foam_v5 (Autodesk Fusion 360 design; units mm, degrees)
Autodesk Fusion 360 part; units mm, degrees
sketch "Sketch1" plane through (0, 0, 0) normal (0, 1, 0) x (1, 0, 0)
  line L0 (0, 0) -> (215.9, 0)
  line L1 (215.9, 0) -> (215.9, 106.3625) construction
  line L2 (215.9, 106.3625) -> (0, 106.3625) construction
  line L3 (0, 106.3625) -> (0, 0)
  line L4 (23, 12) -> (193.9, 12) construction
  line L5 (193.9, 12) -> (193.9, 95.3625) construction
  line L6 (193.9, 95.3625) -> (23, 95.3625) construction
  line L7 (23, 95.3625) -> (23, 12) construction
  circle A0 centre (23, 95.3625) radius 3
  circle A1 centre (23, 12) radius 3
  circle A2 centre (193.9, 12) radius 3
  circle A3 centre (193.9, 95.3625) radius 3
  line L8 (431.8, 0) -> (431.8, 106.3625)
  line L9 (215.9, 0) -> (431.8, 0)
  line L10 (431.8, 106.3625) -> (215.9, 106.3625) construction
  line L11 (215.9, 106.3625) -> (215.9, 0) construction
  line L12 (409.8, 12) -> (409.8, 95.3625) construction
  line L13 (409.8, 95.3625) -> (238.9, 95.3625) construction
  circle A4 centre (409.8, 95.3625) radius 3
  circle A5 centre (238.9, 95.3625) radius 3
  circle A6 centre (409.8, 12) radius 3
  line L14 (238.9, 95.3625) -> (238.9, 12) construction
  line L15 (238.9, 12) -> (409.8, 12) construction
  circle A7 centre (238.9, 12) radius 3
  line L16 (215.9, 106.3625) -> (215.9, 212.725) construction
  line L17 (0, 106.3625) -> (215.9, 106.3625) construction
  line L18 (215.9, 212.725) -> (0, 212.725)
  line L19 (0, 212.725) -> (0, 106.3625)
  line L20 (193.9, 118.3625) -> (193.9, 201.725) construction
  line L21 (193.9, 201.725) -> (23, 201.725) construction
  circle A8 centre (193.9, 201.725) radius 3
  circle A9 centre (23, 201.725) radius 3
  circle A10 centre (193.9, 118.3625) radius 3
  line L22 (23, 201.725) -> (23, 118.3625) construction
  line L23 (23, 118.3625) -> (193.9, 118.3625) construction
  circle A11 centre (23, 118.3625) radius 3
  line L24 (431.8, 106.3625) -> (431.8, 212.725)
  line L25 (215.9, 106.3625) -> (431.8, 106.3625) construction
  line L26 (431.8, 212.725) -> (215.9, 212.725)
  line L27 (215.9, 212.725) -> (215.9, 106.3625) construction
  line L28 (409.8, 118.3625) -> (409.8, 201.725) construction
  line L29 (409.8, 201.725) -> (238.9, 201.725) construction
  circle A12 centre (409.8, 201.725) radius 3
  circle A13 centre (238.9, 201.725) radius 3
  circle A14 centre (409.8, 118.3625) radius 3
  line L30 (238.9, 201.725) -> (238.9, 118.3625) construction
  line L31 (238.9, 118.3625) -> (409.8, 118.3625) construction
  circle A15 centre (238.9, 118.3625) radius 3
  line L32 (33, 190.725) -> (183.9, 190.725)
  line L33 (183.9, 190.725) -> (183.9, 16)
  line L34 (183.9, 16) -> (33, 16)
  line L35 (33, 16) -> (33, 190.725)
  line L36 (248.9, 190.725) -> (399.8, 190.725)
  line L37 (399.8, 190.725) -> (399.8, 16)
  line L38 (399.8, 16) -> (248.9, 16)
  line L39 (248.9, 16) -> (248.9, 190.725)
  point P0 (215.9, 0)
  point P1 (0, 106.3625)
  point P2 (215.9, 106.3625)
  dimension "d35" = 106.3625
  dimension "d36" = 215.9
  dimension "d37" = 23
  dimension "d38" = 11
  dimension "d39" = 12
  dimension "d40" = 22
  dimension "d41" = 6
  dimension "d42" = 6
  dimension "d43" = 6
  dimension "d44" = 6
  dimension "d47" = 215.9
  dimension "d48" = 106.3625
  dimension "d49" = 10
  dimension "d51" = 11
  dimension "d52" = 4
  dimension "d53" = 10
  dimension "d54" = 10
  dimension "d55" = 11
  dimension "d56" = 10
  dimension "d57" = 4
  constraint horizontal L0
  constraint vertical L1
  constraint horizontal L2
  constraint vertical L3
  constraint coincident L0.start L3.end
  constraint horizontal L4
  constraint vertical L5
  constraint horizontal L6
  constraint vertical L7
  constraint coincident L6.end L7.start
  constraint coincident L4.start L7.end
  constraint coincident L4.end L5.start
  constraint coincident L5.end L6.start
  constraint horizontal L32
  constraint vertical L33
  constraint horizontal L34
  constraint vertical L35
  constraint horizontal L36
  constraint vertical L37
  constraint horizontal L38
  constraint vertical L39
  measures "d35" distance of L0.start L2.end
  measures "d36" distance of L0.start P0
  measures "d37" distance of L3 L7
  measures "d38" distance of L2 L6
  measures "d39" distance of L0 L4
  measures "d40" distance of L1 L5
  measures "d41" diameter of A0
  measures "d42" diameter of A1
  measures "d43" diameter of A3
  measures "d44" diameter of A2
  measures "d49" distance of L22.end L35
  measures "d51" distance of L21 L32
  measures "d52" distance of L4 L34
  measures "d53" distance of L5 L33
  measures "d54" distance of L30.end L39
  measures "d55" distance of L29 L36
  measures "d56" distance of L28.end L37
  measures "d57" distance of L14.end L38
extrude "Extrude1" add sketch "Sketch1" along normal blind 2.4
sketch "export" plane through (0, 2.4, 0) normal (0, 1, 0) x (-1, 0, 0)
  circle A0 centre (-23, -12) radius 3
  circle A1 centre (-23, -118.3625) radius 3
  line L0 (-399.8, -16) -> (-248.9, -16)
  line L1 (-248.9, -16) -> (-248.9, -190.725)
  line L2 (-248.9, -190.725) -> (-399.8, -190.725)
  line L3 (-399.8, -190.725) -> (-399.8, -16)
  circle A2 centre (-193.9, -12) radius 3
  circle A3 centre (-409.8, -118.3625) radius 3
  circle A4 centre (-23, -95.3625) radius 3
  circle A5 centre (-238.9, -201.725) radius 3
  circle A6 centre (-409.8, -201.725) radius 3
  circle A7 centre (-238.9, -118.3625) radius 3
  circle A8 centre (-23, -201.725) radius 3
  circle A9 centre (-193.9, -118.3625) radius 3
  line L4 (-183.9, -16) -> (-33, -16)
  line L5 (-33, -16) -> (-33, -190.725)
  line L6 (-33, -190.725) -> (-183.9, -190.725)
  line L7 (-183.9, -190.725) -> (-183.9, -16)
  circle A10 centre (-193.9, -95.3625) radius 3
  circle A11 centre (-193.9, -201.725) radius 3
  circle A12 centre (-409.8, -95.3625) radius 3
  circle A13 centre (-238.9, -12) radius 3
  circle A14 centre (-409.8, -12) radius 3
  circle A15 centre (-238.9, -95.3625) radius 3
  line L8 (-431.8, -212.725) -> (0, -212.725)
  line L9 (0, -212.725) -> (0, 0)
  line L10 (0, 0) -> (-431.8, 0)
  line L11 (-431.8, 0) -> (-431.8, -212.725)
equation "d35 = 8.375 in / 2"
equation "d36 = 17 in / 2"
equation "d42 = d41"
equation "d43 = d41"
equation "d44 = d41"
equation "d51 = d38"
equation "d52 = d51 - 7 mm"
equation "d53 = d49"
equation "d54 = d53"
equation "d55 = d51"
equation "d56 = d54"
equation "d57 = d52"
